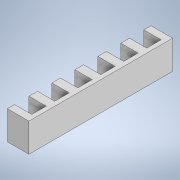
# Autodesk Inventor part: pneunet_approximate_test
Saved by Autodesk Inventor 2021 (Build 250183000, 183)
## iProperties
Created: 2021-03-25
Part Number: pneunet_approximate_test
Material: Generic
Document SubType Name: Modeling
Designer: Charlie
Density: 1 g/cm^3
Appearance: Default
Author: Charlie
Autodesk Inventor part; units mm, degrees
ref_plane "YZ Plane" through (0, 0, 0) normal (1, 0, 0) x (0, 1, 0)
ref_plane "XZ Plane" through (0, 0, 0) normal (0, 1, 0) x (-1, 0, 0)
ref_plane "XY Plane" through (0, 0, 0) normal (0, 0, 1) x (1, 0, 0)
sketch "Sketch1" plane through (0, 0, 0) normal (0, 1, 0) x (-1, 0, 0)
  line L0 (7.5, 50) -> (-7.5, 50)
  line L1 (-7.5, 50) -> (-7.5, -50)
  line L2 (-7.5, -50) -> (7.5, -50)
  line L3 (7.5, -50) -> (7.5, 50) construction
  line L4 (7.5, 50) -> (-7.5, -50) construction
  line L5 (-7.5, 50) -> (7.5, -50) construction
  line L6 (7.5, 50) -> (7.5, 45)
  line L7 (7.5, 35) -> (-4.5, 35)
  line L8 (-4.5, 35) -> (-4.5, 45)
  line L9 (-4.5, 45) -> (7.5, 45)
  line L10 (7.5, 19) -> (-4.5, 19)
  line L11 (-4.5, 19) -> (-4.5, 29)
  line L12 (-4.5, 29) -> (7.5, 29)
  line L13 (7.5, 3) -> (-4.5, 3)
  line L14 (-4.5, 3) -> (-4.5, 13)
  line L15 (-4.5, 13) -> (7.5, 13)
  line L16 (7.5, -13) -> (-4.5, -13)
  line L17 (-4.5, -13) -> (-4.5, -3)
  line L18 (-4.5, -3) -> (7.5, -3)
  line L19 (7.5, -29) -> (-4.5, -29)
  line L20 (-4.5, -29) -> (-4.5, -19)
  line L21 (-4.5, -19) -> (7.5, -19)
  line L22 (7.5, -45) -> (-4.5, -45)
  line L23 (-4.5, -45) -> (-4.5, -35)
  line L24 (-4.5, -35) -> (7.5, -35)
  line L25 (7.5, 35) -> (7.5, 29)
  line L26 (7.5, 19) -> (7.5, 13)
  line L27 (7.5, 3) -> (7.5, -3)
  line L28 (7.5, -13) -> (7.5, -19)
  line L29 (7.5, -29) -> (7.5, -35)
  line L30 (7.5, -45) -> (7.5, -50)
  point P0 (0, 0)
  point P1 (7.5, 0)
  dimension "d0" = 15
  dimension "d1" = 100
  dimension "d4" = 5
  dimension "d5" = 10
  dimension "d6" = 12
  dimension "d9" = 16
  dimension "d14" = 10
  constraints: 62 end point, 5 collinear, 3 midpoint, 3 parallel, 2 perpendicular, 2 point on line, 1 horizontal, 1 vertical, 35 other
  measures "d0" distance of L2.end L1.end
  measures "d1" distance of L1.end L0.end
  measures "d4" distance of L0.start L6.end
  measures "d5" distance of L6.end L7.start
  measures "d6" distance of L7.start L7.end
  measures "d9" distance of L7.start L10.start
  measures "d14" distance of L16.end L17.end
extrude "Extrusion1" add sketch "Sketch1" along normal blind 20
body "Solid1"
